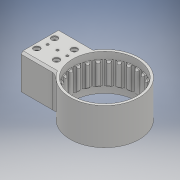
# Autodesk Inventor part: output_housing
Saved by Autodesk Inventor 2017 (Build 210142000, 142)
## iProperties
Created: 2021-02-25
Part Number: output_housing
Material: Generic
Document SubType Name: Modeling
Designer: paulg
Density: 1 g/cm^3
Appearance: Default
Author: paulg
Autodesk Inventor part; units mm, degrees
ref_plane "YZ Plane" through (0, 0, 0) normal (1, 0, 0) x (0, 1, 0)
ref_plane "XZ Plane" through (0, 0, 0) normal (0, 1, 0) x (-1, 0, 0)
ref_plane "XY Plane" through (0, 0, 0) normal (0, 0, 1) x (1, 0, 0)
sketch "Sketch1" plane through (0, 0, 0) normal (0, 0, 1) x (1, 0, 0)
  line L0 (0, 0) -> (31.65, 0) construction
  circle A0 centre (31.65, 0) radius 1.9
  circle A1 centre (0, 0) radius 32.5 construction
  dimension "d0" = 3.8
  dimension "d1" = 31.65
  dimension "d11" = 65
  constraints: 2 centre point, 2 coincident, 2 end point, 1 horizontal
  measures "d0" diameter of A0
  measures "d1" distance of L0.start L0.end
  measures "d11" diameter of A1
extrude "Extrusion1" add sketch "Sketch1" along normal mid plane 23
pattern_circular "Circular Pattern1" count 25 over 360 about axis through (0, 0, -10) along (0, 0, 1) of "Extrusion1"
sketch "Sketch2" plane through (0, 0, 0) normal (0, 0, 1) x (1, 0, 0)
  circle A0 centre (0, 0) radius 32.6
  circle A1 centre (0, 0) radius 35
  dimension "d7" = 65.2
  dimension "d8" = 70
  constraints: 2 centre point, 2 coincident
  measures "d7" diameter of A0
  measures "d8" diameter of A1
extrude "Extrusion2" add sketch "Sketch2" along normal mid plane 37
fillet "Fillet1" radius 1.5 4 edges at (32.5572, 1.6694, 5.75) (32.5572, -1.6694, 5.75) (32.5572, 1.6694, -5.75) (32.5572, -1.6694, -5.75)
pattern_circular "Circular Pattern2" count 25 over 360 about axis through (0, 0, -10) along (0, 0, 1) of "Fillet1"
sketch "Sketch3" plane through (0, 0, 0) normal (0, 0, 1) x (1, 0, 0)
  circle A0 centre (0, 0) radius 35 projected
  line L0 (0, 0) -> (-46.8614, 0) construction
  line L1 (-65, -20) -> (-28.7228, -20)
  line L2 (-28.7228, -20) -> (-28.7228, 20) construction
  line L3 (-28.7228, 20) -> (-65, 20)
  line L4 (-65, 20) -> (-65, -20)
  line L5 (-65, -20) -> (-28.7228, 20) construction
  line L6 (-28.7228, -20) -> (-65, 20) construction
  arc A1 (-28.7228, 20) -> (-28.7228, -20) centre (0, 0) ccw
  dimension "d16" = 65
  dimension "d17" = 40
  constraints: 14 end point, 2 horizontal, 2 midpoint, 2 parallel, 2 point on circle, 1 centre point, 1 coincident, 1 perpendicular, 2 other
  measures "d16" distance from line of point (0, 0) L4
  measures "d17" distance of L3.end L1.start
extrude "Extrusion3" add sketch "Sketch3" along normal up to surface (37 mm away) from surface at -18.5 contours A0 L1 L4 L3
sketch "Sketch4" plane through (0, 0, 0) normal (0, 1, 0) x (-1, 0, 0)
  line L0 (0, 0) -> (0, -11.5)
  line L1 (0, -11.5) -> (-31.5, -11.5)
  line L2 (-31.5, -11.5) -> (-29.5, -9.5)
  line L3 (-29.5, -9.5) -> (-29.5, -11.5)
  line L4 (-32.6, 18.5) -> (32.6, 18.5) projected
  line L5 (32.6, -18.5) -> (-32.6, -18.5) projected
  line L6 (-26.7271, 11.5) -> (-30.0814, 11.5) projected
  line L7 (-30.0814, -11.5) -> (-26.7271, -11.5) projected
  line L8 (-21.2453, 11.5) -> (-26.0116, 11.5) projected
  line L9 (-26.0116, -11.5) -> (-21.2453, -11.5) projected
  line L10 (-14.4286, 11.5) -> (-20.3075, 11.5) projected
  line L11 (-20.3075, -11.5) -> (-14.4286, -11.5) projected
  line L12 (-6.7054, 11.5) -> (-13.3273, 11.5) projected
  line L13 (-13.3273, -11.5) -> (-6.7054, -11.5) projected
  line L14 (1.4392, 11.5) -> (-5.5098, 11.5) projected
  line L15 (-5.5098, -11.5) -> (1.4392, -11.5) projected
  line L16 (9.4934, 11.5) -> (2.654, 11.5) projected
  line L17 (2.654, -11.5) -> (9.4934, -11.5) projected
  line L18 (16.9511, 11.5) -> (10.651, 11.5) projected
  line L19 (10.651, -11.5) -> (16.9511, -11.5) projected
  line L20 (23.3436, 11.5) -> (17.9788, 11.5) projected
  line L21 (17.9788, -11.5) -> (23.3436, -11.5) projected
  line L22 (28.2694, 11.5) -> (24.1768, 11.5) projected
  line L23 (24.1768, -11.5) -> (28.2694, -11.5) projected
  line L24 (31.419, 11.5) -> (28.8558, 11.5) projected
  line L25 (28.8558, -11.5) -> (31.419, -11.5) projected
  line L26 (32.5943, 11.5) -> (31.7217, 11.5) projected
  line L27 (31.7217, -11.5) -> (32.5943, -11.5) projected
  line L28 (31.7217, 11.5) -> (32.5943, 11.5) projected
  line L29 (32.5943, -11.5) -> (31.7217, -11.5) projected
  line L30 (28.8558, 11.5) -> (31.419, 11.5) projected
  line L31 (31.419, -11.5) -> (28.8558, -11.5) projected
  line L32 (24.1768, 11.5) -> (28.2694, 11.5) projected
  line L33 (28.2694, -11.5) -> (24.1768, -11.5) projected
  line L34 (17.9788, 11.5) -> (23.3436, 11.5) projected
  line L35 (23.3436, -11.5) -> (17.9788, -11.5) projected
  line L36 (10.651, 11.5) -> (16.9511, 11.5) projected
  line L37 (16.9511, -11.5) -> (10.651, -11.5) projected
  line L38 (2.654, 11.5) -> (9.4934, 11.5) projected
  line L39 (9.4934, -11.5) -> (2.654, -11.5) projected
  line L40 (-5.5098, 11.5) -> (1.4392, 11.5) projected
  line L41 (1.4392, -11.5) -> (-5.5098, -11.5) projected
  line L42 (-13.3273, 11.5) -> (-6.7054, 11.5) projected
  line L43 (-6.7054, -11.5) -> (-13.3273, -11.5) projected
  line L44 (-20.3075, 11.5) -> (-14.4286, 11.5) projected
  line L45 (-14.4286, -11.5) -> (-20.3075, -11.5) projected
  line L46 (-26.0116, 11.5) -> (-21.2453, 11.5) projected
  line L47 (-21.2453, -11.5) -> (-26.0116, -11.5) projected
  line L48 (-30.0814, 11.5) -> (-26.7271, 11.5) projected
  line L49 (-26.7271, -11.5) -> (-30.0814, -11.5) projected
  line L50 (-32.261, 11.5) -> (-30.5295, 11.5) projected
  line L51 (-30.5295, -11.5) -> (-32.261, -11.5) projected
  line L52 (-32.4136, 11.5) -> (-32.4136, 11.5) projected
  line L53 (-32.4136, -11.5) -> (-32.4136, 11.5) projected
  line L54 (-32.4136, -11.5) -> (-32.4136, -11.5) projected
  line L55 (-32.4136, 11.5) -> (-32.4136, -11.5) projected
  line L56 (-26.7271, -11.5) -> (-26.7271, 11.5) projected
  line L57 (-30.0814, 11.5) -> (-30.0814, -11.5) projected
  line L58 (-21.2453, -11.5) -> (-21.2453, 11.5) projected
  line L59 (-26.0116, 11.5) -> (-26.0116, -11.5) projected
  line L60 (-14.4286, -11.5) -> (-14.4286, 11.5) projected
  line L61 (-20.3075, 11.5) -> (-20.3075, -11.5) projected
  line L62 (-6.7054, -11.5) -> (-6.7054, 11.5) projected
  line L63 (-13.3273, 11.5) -> (-13.3273, -11.5) projected
  line L64 (1.4392, -11.5) -> (1.4392, 11.5) projected
  line L65 (-5.5098, 11.5) -> (-5.5098, -11.5) projected
  line L66 (9.4934, -11.5) -> (9.4934, 11.5) projected
  line L67 (2.654, 11.5) -> (2.654, -11.5) projected
  line L68 (16.9511, -11.5) -> (16.9511, 11.5) projected
  line L69 (10.651, 11.5) -> (10.651, -11.5) projected
  line L70 (23.3436, -11.5) -> (23.3436, 11.5) projected
  line L71 (17.9788, 11.5) -> (17.9788, -11.5) projected
  line L72 (28.2694, -11.5) -> (28.2694, 11.5) projected
  line L73 (24.1768, 11.5) -> (24.1768, -11.5) projected
  line L74 (31.419, -11.5) -> (31.419, 11.5) projected
  line L75 (28.8558, 11.5) -> (28.8558, -11.5) projected
  line L76 (32.5943, -11.5) -> (32.5943, 11.5) projected
  line L77 (31.7217, 11.5) -> (31.7217, -11.5) projected
  line L78 (31.7217, -11.5) -> (31.7217, 11.5) projected
  line L79 (32.5943, 11.5) -> (32.5943, -11.5) projected
  line L80 (28.8558, -11.5) -> (28.8558, 11.5) projected
  line L81 (31.419, 11.5) -> (31.419, -11.5) projected
  line L82 (24.1768, -11.5) -> (24.1768, 11.5) projected
  line L83 (28.2694, 11.5) -> (28.2694, -11.5) projected
  line L84 (17.9788, -11.5) -> (17.9788, 11.5) projected
  line L85 (23.3436, 11.5) -> (23.3436, -11.5) projected
  line L86 (10.651, -11.5) -> (10.651, 11.5) projected
  line L87 (16.9511, 11.5) -> (16.9511, -11.5) projected
  line L88 (2.654, -11.5) -> (2.654, 11.5) projected
  line L89 (9.4934, 11.5) -> (9.4934, -11.5) projected
  line L90 (-5.5098, -11.5) -> (-5.5098, 11.5) projected
  line L91 (1.4392, 11.5) -> (1.4392, -11.5) projected
  line L92 (-13.3273, -11.5) -> (-13.3273, 11.5) projected
  line L93 (-6.7054, 11.5) -> (-6.7054, -11.5) projected
  line L94 (-20.3075, -11.5) -> (-20.3075, 11.5) projected
  line L95 (-14.4286, 11.5) -> (-14.4286, -11.5) projected
  line L96 (-26.0116, -11.5) -> (-26.0116, 11.5) projected
  line L97 (-21.2453, 11.5) -> (-21.2453, -11.5) projected
  line L98 (-30.0814, -11.5) -> (-30.0814, 11.5) projected
  line L99 (-26.7271, 11.5) -> (-26.7271, -11.5) projected
  line L100 (-32.261, -11.5) -> (-32.261, 11.5) projected
  line L101 (-30.5295, 11.5) -> (-30.5295, -11.5) projected
  dimension "d20" = 31.5
  dimension "d21" = 2
  dimension "d22" = 45
  constraints: 8 end point, 1 collinear, 1 parallel, 1 perpendicular, 1 point on line, 1 vertical
  measures "d20" distance of L0.end L1.end
  measures "d21" distance of L2.end L3.end
  measures "d22" angle of L2 L3
revolve "Revolution1" cut sketch "Sketch4" angle 360 about axis through (0, 0, 0) along (0, 0, -1) contours L1 L57 L2 L3 | L1 L101 L2 L57 | L1 L2 L101
mirror "Mirror1" about plane through (0, 0, 0) normal (0, 0, 1) of "Revolution1"
sketch "Sketch5" plane through (-65, -20, 18.5) normal (-1, 0, 0) x (0, 0, 1)
  line L0 (-31.35, 7.2) -> (-5.65, 7.2)
  line L1 (-5.65, 7.2) -> (-5.65, 32.8)
  line L2 (-5.65, 32.8) -> (-31.35, 32.8)
  line L3 (-31.35, 32.8) -> (-31.35, 7.2)
  line L4 (-31.35, 7.2) -> (-5.65, 32.8) construction
  line L5 (-5.65, 7.2) -> (-31.35, 32.8) construction
  line L6 (-31.35, 32.0929) -> (-30.6429, 32.8)
  line L7 (-30.6429, 32.8) -> (-31.35, 33.5071)
  line L8 (-31.35, 33.5071) -> (-32.0571, 32.8)
  line L9 (-32.0571, 32.8) -> (-31.35, 32.0929)
  line L10 (-31.35, 32.0929) -> (-31.35, 33.5071) construction
  line L11 (-30.6429, 32.8) -> (-32.0571, 32.8) construction
  line L12 (-5.65, 32.0929) -> (-6.3571, 32.8)
  line L13 (-6.3571, 32.8) -> (-5.65, 33.5071)
  line L14 (-5.65, 33.5071) -> (-4.9429, 32.8)
  line L15 (-4.9429, 32.8) -> (-5.65, 32.0929)
  line L16 (-5.65, 32.0929) -> (-5.65, 33.5071) construction
  line L17 (-6.3571, 32.8) -> (-4.9429, 32.8) construction
  line L18 (-30.6429, 7.2) -> (-31.35, 6.4929)
  line L19 (-31.35, 6.4929) -> (-32.0571, 7.2)
  line L20 (-32.0571, 7.2) -> (-31.35, 7.9071)
  line L21 (-31.35, 7.9071) -> (-30.6429, 7.2)
  line L22 (-30.6429, 7.2) -> (-32.0571, 7.2) construction
  line L23 (-31.35, 6.4929) -> (-31.35, 7.9071) construction
  line L24 (-6.3571, 7.2) -> (-5.65, 6.4929)
  line L25 (-5.65, 6.4929) -> (-4.9429, 7.2)
  line L26 (-4.9429, 7.2) -> (-5.65, 7.9071)
  line L27 (-5.65, 7.9071) -> (-6.3571, 7.2)
  line L28 (-6.3571, 7.2) -> (-4.9429, 7.2) construction
  line L29 (-5.65, 6.4929) -> (-5.65, 7.9071) construction
  point P0 (-18.5, 20)
  dimension "d24" = 25.6
  dimension "d25" = 25.7
  dimension "d26" = 1
  constraints: 60 end point, 11 parallel, 10 midpoint, 6 equal length, 6 perpendicular, 4 horizontal
  measures "d24" distance of L0.end L1.end
  measures "d25" distance of L0.start L0.end
  measures "d26" distance of L7.end L8.end
extrude "Extrusion4" cut sketch "Sketch5" against normal blind 30
chamfer "Chamfer1" distance 2 angle 45 4 edges at (-46.8614, -20, -18.5) (-46.8614, 20, -18.5) (-46.8614, -20, 18.5) (-46.8614, 20, 18.5)
fillet "Fillet2" radius 10 2 edges at (-28.7228, -20, 0) (-28.7228, 20, 0)
sketch "Sketch6" plane through (0, 0, 18.5) normal (0, 0, 1) x (1, 0, 0)
  circle A0 centre (0, 0) radius 32.6 projected
  arc A1 (-30.0167, -18) -> (-30.0167, 18) centre (0, 0) ccw projected
  line L0 (-65, 18) -> (-30.0167, 18) projected
  line L1 (-65, -18) -> (-65, 18) projected
  line L2 (-30.0167, -18) -> (-65, -18) projected
  line L3 (-65, 12.0929) -> (-35, 12.0929) projected
  line L4 (-35, 12.0929) -> (-35, -12.0929) projected
  line L5 (-65, -12.0929) -> (-35, -12.0929) projected
  line L6 (-65, 12.0929) -> (-65, -12.0929) projected
  line L7 (0, 0) -> (-65, 0)
  line L8 (-40, -9) -> (-60, -9) construction
  line L9 (-60, -9) -> (-60, 9) construction
  line L10 (-60, 9) -> (-40, 9) construction
  line L11 (-40, 9) -> (-40, -9) construction
  line L12 (-40, -9) -> (-60, 9) construction
  line L13 (-60, -9) -> (-40, 9) construction
  point P0 (-50, 0)
  dimension "d33" = 18
  dimension "d34" = 5
  dimension "d35" = 5
  constraints: 14 end point, 4 coincident, 3 midpoint, 2 parallel, 1 horizontal, 1 perpendicular, 1 point on line
  measures "d33" distance of L8.end L9.end
  measures "d34" distance between parallel lines of L1 L9
  measures "d35" distance between parallel lines of L4 L11
hole "Hole1" at (-60, 9, 18.5) at (-40, 9, 18.5) at (-40, -9, 18.5) at (-60, -9, 18.5) direction (0, 0, -1) diameter 3.2 depth 8 tip angle 118 counterbore diameter 6.2 counterbore depth 2.5
chamfer "Chamfer2" distance 1.5 angle 45 4 edges at (-40, 12.1, 16) (-60, 12.1, 16) (-60, -5.9, 16) (-40, -5.9, 16)
mirror "Mirror2" about plane through (0, 0, 0) normal (0, 0, 1) of "Hole1", "Chamfer2"
sketch "Sketch7" plane through (0, 0, 18.5) normal (0, 0, 1) x (1, 0, 0)
  circle A0 centre (-40, -9) radius 3.1 projected
  circle A1 centre (-60, 9) radius 3.1 projected
  circle A2 centre (-40, 9) radius 3.1 projected
  circle A3 centre (-60, -9) radius 3.1 projected
  circle A4 centre (0, 0) radius 32.6 projected
  arc A5 (-30.0167, -18) -> (-30.0167, 18) centre (0, 0) ccw projected
  line L0 (-65, 18) -> (-30.0167, 18) projected
  line L1 (-65, -18) -> (-65, 18) projected
  line L2 (-30.0167, -18) -> (-65, -18) projected
  line L3 (-65, 0) -> (0, 0)
  point P0 (-58, 0)
  point P1 (-48, 0)
  point P2 (-38, 0)
  dimension "d47" = 10
  dimension "d48" = 10
  dimension "d56" = 38
  constraints: 3 point on line, 2 end point, 1 horizontal, 1 midpoint
  measures "d47" distance of point (-48, 0) point (-58, 0)
  measures "d48" distance of point (-48, 0) point (-38, 0)
  measures "d56" distance of point (-38, 0) point (0, 0)
hole "Hole2" at (-58, 0, 18.5) at (-48, 0, 18.5) at (-38, 0, 18.5) direction (0, 0, -1) diameter 2.5 end through all
equation "\"E_\" = 1"
equation "\"Rr_\" = 2"
equation "\"R_\" = 31.5"
body "Solid1"
